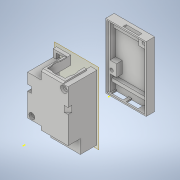
# Autodesk Inventor part: simplemotor
Saved by Autodesk Inventor 2020 (Build 240168000, 168)
## iProperties
Created: 2019-09-09
Part Number: simplemotor
Material: Generic
Document SubType Name: Modeling
Designer: main
Density: 1 g/cm^3
Appearance: Default
Author: main
Autodesk Inventor part; units mm, degrees
ref_plane "YZ Plane" through (0, 0, 0) normal (1, 0, 0) x (0, 1, 0)
ref_plane "XZ Plane" through (0, 0, 0) normal (0, 1, 0) x (-1, 0, 0)
ref_plane "XY Plane" through (0, 0, 0) normal (0, 0, 1) x (1, 0, 0)
sketch "Sketch1" plane through (0, 0, 0) normal (0, 0, 1) x (1, 0, 0)
  line L0 (4.2733, 8.7846) -> (45.3733, 8.7846)
  line L1 (45.3733, 8.7846) -> (45.3733, 74.5846)
  line L2 (45.3733, 74.5846) -> (4.2733, 74.5846)
  line L3 (4.2733, 74.5846) -> (4.2733, 8.7846)
  point P0 (0, 0)
  dimension "d0" = 41.1
  dimension "d1" = 65.8
  constraints: 8 end point, 2 parallel, 1 horizontal, 1 perpendicular
  measures "d0" distance of L1.end L2.end
  measures "d1" distance of L0.end L1.end
extrude "main_body" add sketch "Sketch1" against normal blind 8.6
sketch "Sketch3" plane through (0, 0, 0) normal (0, 0, 1) x (1, 0, 0)
  line L0 (5.5733, 73.2846) -> (44.0733, 73.2846)
  line L1 (44.0733, 73.2846) -> (44.0733, 10.0846)
  line L2 (44.0733, 10.0846) -> (5.5733, 10.0846)
  line L3 (5.5733, 10.0846) -> (5.5733, 73.2846)
  line L4 (4.2733, 74.5846) -> (4.2733, 8.7846) projected
  line L5 (45.3733, 74.5846) -> (4.2733, 74.5846) projected
  line L6 (45.3733, 8.7846) -> (45.3733, 74.5846) projected
  line L7 (4.2733, 8.7846) -> (45.3733, 8.7846) projected
  point P0 (0, 0)
  dimension "d4" = 1.3
  dimension "d5" = 1.3
  dimension "d6" = 1.3
  dimension "d7" = 1.3
  constraints: 8 end point, 2 parallel, 1 horizontal, 1 perpendicular
  measures "d4" distance between parallel lines of L4 L3
  measures "d5" distance between parallel lines of L5 L0
  measures "d6" distance between parallel lines of L6 L1
  measures "d7" distance between parallel lines of L7 L2
extrude "hole_pcb" cut sketch "Sketch3" against normal blind 1.6 contours L0 L1 L2 L3
sketch "Sketch4" plane through (0, 0, -1.6) normal (0, 0, 1) x (1, 0, 0)
  line L0 (7.0733, 73.2846) -> (42.5733, 73.2846)
  line L1 (42.5733, 73.2846) -> (42.5733, 10.0846)
  line L2 (42.5733, 10.0846) -> (7.0733, 10.0846)
  line L3 (7.0733, 10.0846) -> (7.0733, 73.2846)
  line L4 (5.5733, 73.2846) -> (44.0733, 73.2846) projected
  line L5 (44.0733, 10.0846) -> (5.5733, 10.0846) projected
  line L6 (5.5733, 10.0846) -> (5.5733, 73.2846) projected
  line L7 (44.0733, 73.2846) -> (44.0733, 10.0846) projected
  point P0 (0, 0)
  dimension "d10" = 1.5
  dimension "d11" = 1.5
  constraints: 8 end point, 2 collinear, 2 parallel, 1 horizontal, 1 perpendicular
  measures "d10" distance between parallel lines of L6 L3
  measures "d11" distance between parallel lines of L7 L1
extrude "hole_bottom" cut sketch "Sketch4" against normal blind 5.7 contours L0 L1 L2 L3
sketch "Sketch5" plane through (0, 0, -1.6) normal (0, 0, 1) x (1, 0, 0)
  line L0 (13.6943, 26.5086) -> (5.5733, 26.5086)
  line L1 (5.5733, 26.5086) -> (5.5733, 38.5086)
  line L2 (5.5733, 38.5086) -> (13.6943, 38.5086)
  line L3 (13.6943, 38.5086) -> (13.6943, 26.5086)
  line L4 (5.5733, 10.0846) -> (5.5733, 73.2846) projected
  line L5 (44.0733, 10.0846) -> (5.5733, 10.0846) projected
  point P0 (0, 0)
  dimension "d14" = 16.424
  dimension "d15" = 12
  dimension "d16" = 8.121
  constraints: 8 end point, 2 parallel, 1 collinear, 1 horizontal, 1 perpendicular
  measures "d14" distance between parallel lines of L5 L0
  measures "d15" distance of L0.end L1.end
  measures "d16" distance of L1.end L2.end
extrude "support1" add sketch "Sketch5" against normal blind 5.7
sketch "Sketch6" plane through (0, 0, -1.6) normal (0, 0, 1) x (1, 0, 0)
  line L0 (36.4523, 65.6636) -> (44.0733, 65.6636)
  line L1 (44.0733, 65.6636) -> (44.0733, 73.2846)
  line L2 (44.0733, 73.2846) -> (36.4523, 73.2846)
  line L3 (36.4523, 73.2846) -> (36.4523, 65.6636)
  line L4 (5.5733, 73.2846) -> (44.0733, 73.2846) projected
  line L5 (44.0733, 73.2846) -> (44.0733, 10.0846) projected
  point P0 (0, 0)
  dimension "d19" = 7.621
  dimension "d20" = 7.621
  constraints: 8 end point, 2 collinear, 2 parallel, 1 horizontal, 1 perpendicular
  measures "d19" distance of L0.start L0.end
  measures "d20" distance of L2.end L0.start
extrude "support2" add sketch "Sketch6" against normal blind 5.7
sketch "Sketch7" plane through (0, 0, -1.6) normal (0, 0, 1) x (1, 0, 0)
  circle A0 centre (41.2063, 70.3866) radius 1.7
  line L0 (44.0733, 73.2846) -> (44.0733, 10.0846) projected
  line L1 (5.5733, 73.2846) -> (44.0733, 73.2846) projected
  circle A1 centre (8.6943, 30.5086) radius 1.7
  line L2 (5.5733, 10.0846) -> (5.5733, 73.2846) projected
  line L3 (44.0733, 10.0846) -> (5.5733, 10.0846) projected
  point P0 (0, 0)
  dimension "d23" = 2.867
  dimension "d24" = 2.898
  dimension "d25" = 3.4
  dimension "d26" = 3.121
  dimension "d27" = 20.424
  dimension "d28" = 3.4
  constraints: 2 centre point
  measures "d23" distance from line of L0 A0.centre
  measures "d24" distance from line of L1 A0.centre
  measures "d25" diameter of A0
  measures "d26" distance from line of L2 A1.centre
  measures "d27" distance from line of L3 A1.centre
  measures "d28" diameter of A1
sketch "Sketch9" plane through (4.2733, 8.7846, 0) normal (0, -1, 0) x (1, 0, 0)
  line L0 (4.009, -1.6) -> (16.009, -1.6)
  line L1 (16.009, -1.6) -> (16.009, -7.3)
  line L2 (16.009, -7.3) -> (4.009, -7.3)
  line L3 (4.009, -7.3) -> (4.009, -1.6)
  line L4 (0, 0) -> (41.1, 0) projected
  line L5 (1.3, 0) -> (1.3, -1.6) projected
  line L6 (19.249, -1.6) -> (31.249, -1.6)
  line L7 (31.249, -1.6) -> (31.249, -7.3)
  line L8 (31.249, -7.3) -> (19.249, -7.3)
  line L9 (19.249, -7.3) -> (19.249, -1.6)
  point P0 (-4.2733, 0)
  dimension "d35" = 1.6
  dimension "d36" = 5.7
  dimension "d37" = 12
  dimension "d38" = 2.709
  dimension "d39" = 17.949
  constraints: 16 end point, 4 parallel, 3 collinear, 2 horizontal, 2 perpendicular
  measures "d35" distance between parallel lines of L4 L0
  measures "d36" distance of L2.end L0.start
  measures "d37" distance of L1.end L2.end
  measures "d38" distance between parallel lines of L5 L3
  measures "d39" distance between parallel lines of L5 L9
extrude "j1_j2_holes" cut sketch "Sketch9" against normal blind 1.3
sketch "Sketch10" plane through (4.2733, 74.5846, 0) normal (0, 1, 0) x (1, 0, 0)
  line L0 (15.979, 1.6) -> (31.979, 1.6)
  line L1 (31.979, 1.6) -> (31.979, 4.8)
  line L2 (31.979, 4.8) -> (15.979, 4.8)
  line L3 (15.979, 4.8) -> (15.979, 1.6)
  line L4 (16.009, 1.6) -> (4.009, 1.6) projected
  line L5 (1.3, 0) -> (1.3, 1.6) projected
  point P0 (-4.2733, 0)
  dimension "d42" = 3.2
  dimension "d43" = 16
  dimension "d44" = 14.679
  constraints: 8 end point, 2 parallel, 1 collinear, 1 horizontal, 1 perpendicular
  measures "d42" distance of L2.end L0.start
  measures "d43" distance of L1.end L2.end
  measures "d44" distance between parallel lines of L3 L5
extrude "j3_hole" cut sketch "Sketch10" against normal blind 1.3
sketch "Sketch11" plane through (0, 0, -7.3) normal (0, 0, 1) x (1, 0, 0)
  line L0 (7.0733, 18.5846) -> (42.5733, 18.5846)
  line L1 (42.5733, 18.5846) -> (42.5733, 22.0846)
  line L2 (42.5733, 22.0846) -> (7.0733, 22.0846)
  line L3 (7.0733, 22.0846) -> (7.0733, 18.5846)
  line L4 (7.0733, 10.0846) -> (7.0733, 26.5086) projected
  line L5 (42.5733, 65.6636) -> (42.5733, 10.0846) projected
  line L6 (44.0733, 10.0846) -> (5.5733, 10.0846) projected
  point P0 (0, 0)
  dimension "d47" = 8.5
  dimension "d48" = 12
  constraints: 8 end point, 2 collinear, 2 parallel, 1 horizontal, 1 perpendicular
  measures "d47" distance between parallel lines of L0 L6
  measures "d48" distance between parallel lines of L6 L2
extrude "stifness_beam_1" add sketch "Sketch11" along normal blind 3.7 contours L3 L2 L1 L0
sketch "Sketch12" plane through (0, 0, -7.3) normal (0, 0, 1) x (1, 0, 0)
  line L0 (36.4523, 73.2846) -> (7.0733, 73.2846)
  line L1 (7.0733, 73.2846) -> (7.0733, 65.6636)
  line L2 (7.0733, 65.6636) -> (36.4523, 65.6636)
  line L3 (36.4523, 65.6636) -> (36.4523, 73.2846)
  line L4 (36.4523, 73.2846) -> (36.4523, 65.6636) projected
  line L5 (7.0733, 38.5086) -> (7.0733, 73.2846) projected
  line L6 (5.5733, 73.2846) -> (44.0733, 73.2846) projected
  line L7 (36.4523, 65.6636) -> (42.5733, 65.6636) projected
  point P0 (0, 0)
  constraints: 8 end point, 4 collinear, 2 parallel, 1 horizontal, 1 perpendicular
extrude "stifness_beam_2" add sketch "Sketch12" along normal blind 2.5
sketch "Sketch13" plane through (0, 0, -8.6) normal (0, 0, -1) x (-1, 0, 0)
  point P0 (0, 0)
ref_plane "Work Plane1" through (0, 0, 50) normal (0, 0, 1) x (1, 0, 0)
sketch "Sketch15" plane through (0, 0, 50) normal (0, 0, 1) x (1, 0, 0)
  line L0 (45.3733, 74.5846) -> (4.2733, 74.5846)
  line L1 (4.2733, 74.5846) -> (4.2733, 8.7846)
  line L2 (4.2733, 8.7846) -> (45.3733, 8.7846)
  line L3 (45.3733, 8.7846) -> (45.3733, 74.5846)
  line L4 (45.3733, 8.7846) -> (45.3733, 74.5846) projected
  line L5 (45.3733, 74.5846) -> (4.2733, 74.5846) projected
  line L6 (4.2733, 74.5846) -> (4.2733, 8.7846) projected
  line L7 (4.2733, 8.7846) -> (45.3733, 8.7846) projected
  point P0 (0, 0)
  constraints: 8 end point, 4 collinear, 2 parallel, 1 horizontal, 1 perpendicular
extrude "Extrusion12" add sketch "Sketch15" along normal blind 29.3
sketch "Sketch16" plane through (0, 0, 50) normal (0, 0, 1) x (1, 0, 0)
  line L0 (7.0733, 73.2846) -> (42.5733, 73.2846)
  line L1 (42.5733, 73.2846) -> (42.5733, 10.0846)
  line L2 (42.5733, 10.0846) -> (7.0733, 10.0846)
  line L3 (7.0733, 10.0846) -> (7.0733, 73.2846)
  line L4 (7.0733, 10.0846) -> (7.0733, 26.5086) projected
  line L5 (42.5733, 10.0846) -> (35.5223, 10.0846) projected
  line L6 (42.5733, 65.6636) -> (42.5733, 10.0846) projected
  line L7 (7.0733, 73.2846) -> (20.2523, 73.2846) projected
  point P0 (0, 0)
  constraints: 8 end point, 4 collinear, 2 parallel, 1 horizontal, 1 perpendicular
extrude "Extrusion13" cut sketch "Sketch16" along normal blind 28
sketch "Sketch17" plane through (0, 0, 50) normal (0, 0, -1) x (-1, 0, 0)
  line L0 (-42.5733, 27.5846) -> (-44.2733, 27.5846)
  line L1 (-44.2733, 27.5846) -> (-44.2733, 45.2846)
  line L2 (-44.2733, 45.2846) -> (-42.5733, 45.2846)
  line L3 (-42.5733, 45.2846) -> (-42.5733, 27.5846)
  line L4 (-42.5733, 10.0846) -> (-42.5733, 73.2846) projected
  line L5 (-7.0733, 10.0846) -> (-42.5733, 10.0846) projected
  line L6 (-42.5733, 73.2846) -> (-7.0733, 73.2846) projected
  point P0 (0, 0)
  dimension "d68" = 1.7
  dimension "d69" = 17.5
  dimension "d70" = 28
  constraints: 8 end point, 2 parallel, 1 collinear, 1 horizontal, 1 perpendicular
  measures "d68" distance of L0.start L0.end
  measures "d69" distance between parallel lines of L5 L0
  measures "d70" distance between parallel lines of L6 L2
extrude "Extrusion14" cut sketch "Sketch17" against normal blind 28
sketch "Sketch18" plane through (0, 0, 50) normal (0, 0, 1) x (1, 0, 0)
  line L0 (36.4523, 65.6636) -> (42.5733, 65.6636)
  line L1 (42.5733, 65.6636) -> (42.5733, 73.2846)
  line L2 (42.5733, 73.2846) -> (36.4523, 73.2846)
  line L3 (36.4523, 73.2846) -> (36.4523, 65.6636)
  line L4 (42.5733, 73.2846) -> (42.5733, 45.2846) projected
  line L5 (7.0733, 73.2846) -> (42.5733, 73.2846) projected
  line L6 (36.4523, 73.2846) -> (36.4523, 65.6636) projected
  line L7 (36.4523, 65.6636) -> (42.5733, 65.6636) projected
  line L8 (11.7943, 26.5086) -> (7.0733, 26.5086)
  line L9 (7.0733, 26.5086) -> (7.0733, 34.5086)
  line L10 (7.0733, 34.5086) -> (11.7943, 34.5086)
  line L11 (11.7943, 34.5086) -> (11.7943, 26.5086)
  line L12 (7.0733, 10.0846) -> (7.0733, 73.2846) projected
  line L13 (7.0733, 26.5086) -> (13.6943, 26.5086) projected
  circle A0 centre (8.6943, 30.5086) radius 1.6 projected
  point P0 (0, 0)
  dimension "d73" = 4
  dimension "d74" = 3.1
  constraints: 16 end point, 6 collinear, 4 parallel, 2 horizontal, 2 perpendicular
  measures "d73" distance from line of A0.centre L10
  measures "d74" distance from line of L11 A0.centre
extrude "Extrusion15" add sketch "Sketch18" along normal blind 28 contours L3 L2 L1 L0 | L10 L11 L8 L9 | A0
extrude "Extrusion16" cut sketch "Sketch7" along normal blind 100 and the other way blind 10 contours A0 | A1
sketch "Sketch19" plane through (0, 0, -8.6) normal (0, 0, -1) x (-1, 0, 0)
  circle A0 centre (-8.6943, 30.5086) radius 3
  circle A1 centre (-8.6943, 30.5086) radius 1.7 projected
  circle A2 centre (-41.2063, 70.3866) radius 3.5
  circle A3 centre (-41.2063, 70.3866) radius 1.7 projected
  point P0 (0, 0)
  dimension "d81" = 6
  dimension "d82" = 7
  constraints: 2 centre point, 2 concentric
  measures "d81" diameter of A0
  measures "d82" diameter of A2
extrude "Extrusion17" cut sketch "Sketch19" along normal blind 2.5 from surface at -87.9
sketch "Sketch21" plane through (4.2733, 8.7846, 50) normal (0, -1, 0) x (1, 0, 0)
  line L0 (18.479, 1.8) -> (29.479, 1.8)
  line L1 (29.479, 1.8) -> (29.479, 8.6)
  line L2 (29.479, 8.6) -> (18.479, 8.6)
  line L3 (18.479, 8.6) -> (18.479, 1.8)
  line L4 (0, 0) -> (41.1, 0) projected
  line L5 (1.3, -50) -> (1.3, -51.6) projected
  point P0 (-4.2733, -50)
  dimension "d92" = 1.8
  dimension "d93" = 6.8
  dimension "d94" = 11
  dimension "d95" = 17.179
  constraints: 8 end point, 2 parallel, 1 horizontal, 1 perpendicular
  measures "d92" distance between parallel lines of L4 L0
  measures "d93" distance of L2.end L0.start
  measures "d94" distance of L1.end L2.end
  measures "d95" distance between parallel lines of L3 L5
extrude "Extrusion19" cut sketch "Sketch21" against normal blind 1.3
sketch "Sketch22" plane through (0, 0, -7.3) normal (0, 0, 1) x (1, 0, 0)
  point P0 (0, 0)
sketch "Sketch23" plane through (0, 0, 50) normal (0, 0, 1) x (1, 0, 0)
  point P0 (0, 0)
sketch "Sketch24" plane through (0, 0, 50) normal (0, 0, 1) x (1, 0, 0)
  line L0 (18.8663, 65.5996) -> (4.2733, 65.5996)
  line L1 (4.2733, 65.5996) -> (4.2733, 74.5846)
  line L2 (4.2733, 74.5846) -> (18.8663, 74.5846)
  line L3 (18.8663, 74.5846) -> (18.8663, 65.5996)
  line L4 (19.2523, 74.5846) -> (4.2733, 74.5846)
  line L5 (4.2733, 74.5846) -> (4.2733, 8.7846) projected
  line L6 (45.3733, 74.5846) -> (4.2733, 74.5846) projected
  point P0 (0, 0)
  dimension "d98" = 8.985
  dimension "d110" = 14.593
  constraints: 10 end point, 2 collinear, 2 parallel
  measures "d98" distance of L2.end L0.start
  measures "d110" distance between parallel lines of L1 L3
extrude "Extrusion20" add sketch "Sketch24" along normal blind 29.3
sketch "Sketch20" plane through (4.2733, 74.5846, 50) normal (0, 1, 0) x (1, 0, 0)
  line L0 (32.979, -5.7) -> (14.979, -5.7)
  line L1 (14.979, -5.7) -> (14.979, 0)
  line L2 (14.979, 0) -> (32.979, 0)
  line L3 (32.979, 0) -> (32.979, -5.7)
  line L4 (41.1, 0) -> (0, 0) projected
  line L5 (41.1, 0) -> (41.1, -29.3) projected
  line L6 (1.3, 50) -> (1.3, 51.6) projected
  point P0 (-4.2733, 50)
  dimension "d86" = 18
  dimension "d88" = 13.679
  dimension "d89" = 5.7
  constraints: 8 end point, 2 parallel, 1 collinear, 1 horizontal, 1 perpendicular
  measures "d86" distance of L0.start L0.end
  measures "d88" distance between parallel lines of L1 L6
  measures "d89" distance of L2.end L0.start
extrude "Extrusion18" cut sketch "Sketch20" against normal blind 12
sketch "Sketch25" plane through (0, 0, 79.3) normal (0, 0, 1) x (1, 0, 0)
  line L0 (18.2163, 66.8996) -> (4.2733, 66.8996)
  line L1 (4.2733, 66.8996) -> (4.2733, 74.5846)
  line L2 (4.2733, 74.5846) -> (18.2163, 74.5846)
  line L3 (18.2163, 74.5846) -> (18.2163, 66.8996)
  line L4 (4.2733, 74.5846) -> (4.2733, 65.6496) projected
  line L5 (19.8663, 74.5846) -> (4.2733, 74.5846) projected
  line L6 (5.5733, 10.0846) -> (5.5733, 73.2846) projected
  line L7 (5.5733, 73.2846) -> (44.0733, 73.2846) projected
  point P0 (0, 0)
  dimension "d101" = 12.643
  dimension "d102" = 6.385
  constraints: 8 end point, 2 collinear, 2 parallel, 1 horizontal, 1 perpendicular
  measures "d101" distance between parallel lines of L6 L3
  measures "d102" distance between parallel lines of L7 L0
extrude "Extrusion21" cut sketch "Sketch25" against normal blind 25.9
sketch "Sketch26" plane through (0, 0, 53.4) normal (0, 0, 1) x (1, 0, 0)
  line L0 (18.2163, 66.8996) -> (7.5163, 66.8996)
  line L1 (7.5163, 66.8996) -> (7.5163, 72.3496)
  line L2 (7.5163, 72.3496) -> (18.2163, 72.3496)
  line L3 (18.2163, 72.3496) -> (18.2163, 66.8996)
  line L4 (18.2163, 66.8996) -> (4.2733, 66.8996) projected
  line L5 (18.2163, 74.5846) -> (18.2163, 66.8996) projected
  point P0 (0, 0)
  dimension "d105" = 5.45
  dimension "d106" = 10.7
  constraints: 8 end point, 2 collinear, 2 parallel, 1 horizontal, 1 perpendicular
  measures "d105" distance of L0.end L1.end
  measures "d106" distance of L1.end L2.end
extrude "Extrusion22" cut sketch "Sketch26" against normal blind 3.4
sketch "Sketch27" plane through (0, 0, 50) normal (0, 0, 1) x (1, 0, 0)
  line L0 (18.8663, 27.2796) -> (7.0733, 27.2796)
  line L1 (7.0733, 27.2796) -> (7.0733, 10.0846)
  line L2 (7.0733, 10.0846) -> (18.8663, 10.0846)
  line L3 (18.8663, 10.0846) -> (18.8663, 27.2796)
  line L4 (7.0733, 10.0846) -> (7.0733, 26.5086) projected
  line L5 (42.5733, 10.0846) -> (7.0733, 10.0846) projected
  line L6 (5.5733, 10.0846) -> (5.5733, 73.2846) projected
  point P0 (0, 0)
  dimension "d111" = 17.195
  dimension "d112" = 13.293
  constraints: 8 end point, 2 collinear, 2 parallel, 1 horizontal, 1 perpendicular
  measures "d111" distance between parallel lines of L2 L0
  measures "d112" distance between parallel lines of L6 L3
extrude "Extrusion23" add sketch "Sketch27" along normal blind 29.3
sketch "Sketch28" plane through (0, 0, 79.3) normal (0, 0, 1) x (1, 0, 0)
  point P0 (0, 0)
sketch "Sketch29" plane through (0, 0, 79.3) normal (0, 0, 1) x (1, 0, 0)
  line L0 (18.2163, 26.6296) -> (4.2733, 26.6296)
  line L1 (4.2733, 26.6296) -> (4.2733, 8.7846)
  line L2 (4.2733, 8.7846) -> (18.2163, 8.7846)
  line L3 (18.2163, 8.7846) -> (18.2163, 26.6296)
  line L4 (4.2733, 66.8996) -> (4.2733, 8.7846) projected
  line L5 (4.2733, 8.7846) -> (45.3733, 8.7846) projected
  line L6 (18.8663, 27.2796) -> (11.7943, 27.2796) projected
  line L7 (18.8663, 10.0846) -> (18.8663, 27.2796) projected
  point P0 (0, 0)
  dimension "d169" = 0.65
  dimension "d170" = 0.65
  constraints: 8 end point, 2 collinear, 2 parallel, 1 horizontal, 1 perpendicular
  measures "d169" distance between parallel lines of L6 L0
  measures "d170" distance between parallel lines of L7 L3
extrude "Extrusion24" cut sketch "Sketch29" against normal blind 25.9
sketch "Sketch30" plane through (0, 0, 53.4) normal (0, 0, 1) x (1, 0, 0)
  point P0 (0, 0)
sketch "Sketch31" plane through (0, 0, 53.4) normal (0, 0, 1) x (1, 0, 0)
  line L0 (7.5163, 21.1796) -> (18.2163, 21.1796)
  line L1 (18.2163, 21.1796) -> (18.2163, 26.6296)
  line L2 (18.2163, 26.6296) -> (7.5163, 26.6296)
  line L3 (7.5163, 26.6296) -> (7.5163, 21.1796)
  line L4 (4.2733, 26.6296) -> (18.2163, 26.6296) projected
  line L5 (18.2163, 26.6296) -> (18.2163, 8.7846) projected
  point P0 (0, 0)
  point P1 (7.0733, 26.5796)
  point P2 (18.5663, 10.0846)
  point P3 (18.2163, 8.7846)
  dimension "d119" = 5.45
  dimension "d120" = 10.7
  constraints: 8 end point, 2 horizontal, 2 parallel, 1 perpendicular, 1 vertical, 2 other
  measures "d119" distance of L2.end L0.start
  measures "d120" distance of L0.start L0.end
extrude "Extrusion25" cut sketch "Sketch31" against normal blind 3.4
sketch "Sketch33" plane through (18.8663, 10.0846, 50) normal (1, 0, 0) x (0, 0, -1)
  line L0 (-29.3, 17.145) -> (-24.3, 17.145)
  line L1 (-24.3, 17.145) -> (-24.3, 12.145)
  line L2 (-24.3, 12.145) -> (-29.3, 12.145)
  line L3 (-29.3, 12.145) -> (-29.3, 17.145)
  line L4 (-29.3, 0) -> (-29.3, 17.145) projected
  line L5 (-7, 17.145) -> (-28, 17.145) projected
  point P0 (50, -10.0846)
  dimension "d126" = 5
  dimension "d127" = 5
  constraints: 8 end point, 2 collinear, 2 parallel, 1 horizontal, 1 perpendicular
  measures "d126" distance of L1.end L2.end
  measures "d127" distance of L0.end L1.end
extrude "Extrusion27" add sketch "Sketch33" along normal blind 24.557
sketch "Sketch34" plane through (18.8663, 10.0846, 50) normal (1, 0, 0) x (0, 0, -1)
  line L0 (0, 17.195) -> (-28, 17.195)
  line L1 (-28, 17.195) -> (-28, 17.145)
  line L2 (-28, 17.145) -> (0, 17.145)
  line L3 (0, 17.145) -> (0, 17.195)
  line L4 (0, 17.195) -> (-28, 17.195) projected
  line L5 (0, 0) -> (0, 17.195) projected
  line L6 (-28, 17.145) -> (-24.3, 17.145) projected
  line L7 (-28, 17.145) -> (-28, 17.195) projected
  point P0 (50, -10.0846)
  constraints: 8 end point, 4 collinear, 2 parallel, 1 horizontal, 1 perpendicular
extrude "Extrusion28" cut sketch "Sketch34" against normal up to surface (7.072 mm away)
sketch "Sketch35" plane through (0, 0, 79.3) normal (0, 0, 1) x (1, 0, 0)
  point P0 (0, 0)
sketch "Sketch36" plane through (0, 0, 79.3) normal (0, 0, 1) x (1, 0, 0)
  point P0 (0, 0)
sketch "Sketch37" plane through (0, 0, 79.3) normal (0, 0, 1) x (1, 0, 0)
  line L0 (6.9912, 27.5586) -> (5.288, 30.5086)
  line L1 (5.288, 30.5086) -> (6.9912, 33.4586)
  line L2 (6.9912, 33.4586) -> (10.3975, 33.4586)
  line L3 (10.3975, 33.4586) -> (12.1007, 30.5086)
  line L4 (12.1007, 30.5086) -> (10.3975, 27.5586)
  line L5 (10.3975, 27.5586) -> (6.9912, 27.5586)
  line L6 (4.2733, 26.6296) -> (18.2163, 26.6296) projected
  circle A0 centre (8.6943, 30.5086) radius 2.95 construction
  circle A1 centre (8.6943, 30.5086) radius 1.7 projected
  line L7 (39.5032, 67.4366) -> (37.8, 70.3866)
  line L8 (37.8, 70.3866) -> (39.5032, 73.3366)
  line L9 (39.5032, 73.3366) -> (42.9095, 73.3366)
  line L10 (42.9095, 73.3366) -> (44.6127, 70.3866)
  line L11 (44.6127, 70.3866) -> (42.9095, 67.4366)
  line L12 (42.9095, 67.4366) -> (39.5032, 67.4366)
  line L13 (45.3733, 74.5846) -> (18.2163, 74.5846) projected
  circle A2 centre (41.2063, 70.3866) radius 2.95 construction
  circle A3 centre (41.2063, 70.3866) radius 1.7 projected
  point P0 (0, 0)
  point P1 (8.6943, 30.5086)
  point P2 (19.1163, 26.5796)
  dimension "d132" = 5.9
  dimension "d133" = 5.9
  constraints: 24 end point, 6 tangent, 2 centre point, 2 concentric, 1 horizontal, 1 parallel, 27 other
  measures "d132" distance between parallel lines of L2 L5
  measures "d133" distance between parallel lines of L9 L12
extrude "Extrusion29" cut sketch "Sketch37" along normal blind 3 from surface at -87.9
chamfer "Chamfer2" distance 7 angle 45 2 edges at (39.5128, 65.6636, 78) (36.4523, 69.4741, 78)
sketch "Sketch38" plane through (42.5733, 45.2846, 50) normal (-1, 0, 0) x (0, 0, 1)
  line L0 (28, 0) -> (24, 0)
  line L1 (24, 0) -> (24, 5)
  line L2 (24, 5) -> (28, 5)
  line L3 (28, 5) -> (28, 0)
  line L4 (0, 0) -> (28, 0) projected
  line L5 (28, 0) -> (28, 13.379) projected
  point P0 (-50, -45.2846)
  dimension "d142" = 5
  dimension "d143" = 4
  constraints: 8 end point, 2 collinear, 2 parallel, 1 horizontal, 1 perpendicular
  measures "d142" distance of L0.end L1.end
  measures "d143" distance of L1.end L2.end
extrude "Extrusion30" add sketch "Sketch38" along normal blind 35.5
sketch "Sketch39" plane through (7.0733, 34.5086, 50) normal (0, 1, 0) x (1, 0, 0)
  line L0 (0, -24) -> (4.721, -24)
  line L1 (4.721, -24) -> (4.721, -28)
  line L2 (4.721, -28) -> (0, -28)
  line L3 (0, -28) -> (0, -24)
  line L4 (4.721, 0) -> (4.721, -28) projected
  line L5 (0, -28) -> (0, 0) projected
  line L6 (4.721, -28) -> (0, -28) projected
  point P0 (-7.0733, 50)
  dimension "d146" = 4
  constraints: 8 end point, 3 collinear, 2 parallel, 1 horizontal, 1 perpendicular
  measures "d146" distance of L0.end L1.end
extrude "Extrusion31" add sketch "Sketch39" along normal blind 32
sketch "Sketch40" plane through (11.7943, 27.2296, 78) normal (1, 0, 0) x (0, 0, -1)
  line L0 (0, 0) -> (0, 6)
  line L1 (0, 6) -> (6, 0)
  line L2 (6, 0) -> (0, 0)
  line L3 (0, 0) -> (0, 18.055) projected
  line L4 (28, 0) -> (0, 0) projected
  point P0 (78, -27.2296)
  point P1 (0, 0.05)
  dimension "d149" = 6
  dimension "d150" = 6
  constraints: 6 end point, 2 collinear
  measures "d149" distance of L0.start L0.end
  measures "d150" distance of L1.end L0.start
extrude "Extrusion32" add sketch "Sketch40" along normal up to surface (7.072 mm away)
sketch "Sketch41" plane through (0, 0, 78) normal (0, 0, -1) x (-1, 0, 0)
  point P0 (0, 0)
sketch "Sketch42" plane through (0, 0, 78) normal (0, 0, -1) x (-1, 0, 0)
  point P0 (0, 0)
sketch "Sketch43" plane through (0, 0, 78) normal (0, 0, -1) x (-1, 0, 0)
  point P0 (0, 0)
sketch "Sketch44" plane through (0, 0, 78) normal (0, 0, -1) x (-1, 0, 0)
  line L0 (-20.3663, 10.0846) -> (-18.8663, 10.0846)
  line L1 (-18.8663, 10.0846) -> (-18.8663, 27.2296)
  line L2 (-18.8663, 27.2296) -> (-20.3663, 27.2296)
  line L3 (-20.3663, 27.2296) -> (-20.3663, 10.0846)
  line L4 (-18.8663, 27.2296) -> (-18.8663, 33.2296) projected
  line L5 (-18.8663, 10.0846) -> (-42.5733, 10.0846) projected
  line L6 (-11.7943, 27.2296) -> (-18.8663, 27.2296) projected
  point P0 (0, 0)
  point P1 (-18.8663, 22.2296)
  point P2 (-19.2163, 10.0846)
  point P3 (-18.2163, 27.2296)
  dimension "d153" = 1.5
  constraints: 8 end point, 3 collinear, 2 parallel, 1 horizontal, 1 perpendicular
  measures "d153" distance between parallel lines of L3 L1
extrude "Extrusion33" add sketch "Sketch44" along normal blind 12
sketch "Sketch45" plane through (0, 0, 53.4) normal (0, 0, 1) x (1, 0, 0)
  line L0 (18.2163, 21.1796) -> (18.2163, 8.7846)
  line L1 (18.2163, 8.7846) -> (15.2163, 8.7846)
  line L2 (15.2163, 8.7846) -> (18.2163, 21.1796)
  line L3 (18.2163, 8.7846) -> (4.2733, 8.7846) projected
  line L4 (18.2163, 21.1796) -> (18.2163, 8.7846) projected
  line L5 (18.2163, 21.1796) -> (7.5163, 21.1796) projected
  point P0 (0, 0)
  point P1 (19.2163, 10.0846)
  point P2 (19.1163, 21.1296)
  dimension "d156" = 3
  constraints: 4 end point, 1 collinear, 6 other
  measures "d156" distance of L1.start L1.end
extrude "Extrusion34" add sketch "Sketch45" along normal up to surface (25.9 mm away)
sketch "Sketch46" plane through (0, 0, 50) normal (0, 0, -1) x (-1, 0, 0)
  line L0 (-42.5733, 27.5846) -> (-42.9733, 27.5846)
  line L1 (-42.9733, 27.5846) -> (-42.9733, 10.0846)
  line L2 (-42.9733, 10.0846) -> (-42.5733, 10.0846)
  line L3 (-42.5733, 10.0846) -> (-42.5733, 27.5846)
  line L4 (-42.5733, 10.0846) -> (-42.5733, 27.5846) projected
  line L5 (-42.5733, 27.5846) -> (-44.2733, 27.5846) projected
  line L6 (-18.8663, 10.0846) -> (-42.5733, 10.0846) projected
  point P0 (0, 0)
  dimension "d159" = 0.4
  constraints: 8 end point, 3 collinear, 2 parallel, 1 horizontal, 1 perpendicular
  measures "d159" distance between parallel lines of L3 L1
extrude "Extrusion35" cut sketch "Sketch46" against normal blind 16
sketch "Sketch47" plane through (42.5733, 50.2846, 78) normal (0, 1, 0) x (1, 0, 0)
  line L0 (0, 4) -> (-4, 4)
  line L1 (-4, 4) -> (-4, 0)
  line L2 (-4, 0) -> (0, 0)
  line L3 (0, 0) -> (0, 4)
  line L4 (0, 4) -> (0, 0) projected
  line L5 (0, 0) -> (-30.779, 0) projected
  line L6 (0, 4) -> (-30.779, 4) projected
  point P0 (-42.5733, 78)
  constraints: 8 end point, 3 collinear, 2 parallel, 2 perpendicular, 1 horizontal
extrude "Extrusion36" add sketch "Sketch47" along normal up to surface (15.379 mm away)
sketch "Sketch48" plane through (44.9733, 50.2846, 79.3) normal (0, 1, 0) x (1, 0, 0)
  line L0 (0.4, 4) -> (0.4, 0)
  line L1 (0.4, 0) -> (-3.6, 0)
  line L2 (-3.6, 0) -> (0.4, 4)
  line L3 (0.4, 0) -> (-26.757, 0) projected
  line L4 (0.4, 29.3) -> (0.4, 0) projected
  line L5 (-26.757, 0) -> (-40.7, 0) projected
  line L6 (-40.7, 0) -> (-40.7, 25.9) projected
  line L7 (-36.7, 0) -> (-40.7, 4)
  line L8 (-40.7, 4) -> (-40.7, 0)
  line L9 (-40.7, 0) -> (-36.7, 0)
  point P0 (-44.9733, 79.3)
  point P1 (-36.7, 0)
  dimension "d164" = 4
  constraints: 12 end point, 4 collinear, 3 perpendicular
  measures "d164" distance of L0.end L1.end
extrude "Extrusion38" cut sketch "Sketch48" along normal blind 6
sketch "Sketch49" plane through (20.3663, 10.0846, 78) normal (0, 1, 0) x (1, 0, 0)
  line L0 (22.607, 0) -> (-1.5, 0)
  line L1 (-1.5, 0) -> (-1.5, 12.5)
  line L2 (-1.5, 12.5) -> (22.607, 12.5)
  line L3 (22.607, 12.5) -> (22.607, 0)
  line L4 (22.607, 28) -> (22.607, 12) projected
  line L5 (-1.5, 28) -> (-1.5, 12) projected
  line L6 (-1.5, 28) -> (22.607, 28) projected
  line L7 (0, 0) -> (22.207, 0) projected
  point P0 (-20.3663, 78)
  dimension "d171" = 15.5
  constraints: 8 end point, 3 collinear, 2 parallel, 1 horizontal, 1 perpendicular
  measures "d171" distance between parallel lines of L6 L2
extrude "Extrusion39" add sketch "Sketch49" along normal blind 14 from surface at 0 contours L0 L1 L2 L3
sketch "Sketch52" plane through (4.2733, 8.7846, 50) normal (0, -1, 0) x (1, 0, 0)
  line L0 (10.943, 29.3) -> (41.1, 29.3)
  line L1 (41.1, 29.3) -> (41.1, 16.8)
  line L2 (41.1, 16.8) -> (10.943, 16.8)
  line L3 (10.943, 16.8) -> (10.943, 29.3)
  line L4 (10.943, 29.3) -> (41.1, 29.3) projected
  line L5 (10.943, 3.4) -> (10.943, 29.3) projected
  line L6 (41.1, 0) -> (41.1, 29.3) projected
  line L7 (14.593, 15.5) -> (38.7, 15.5) projected
  point P0 (-4.2733, -50)
  dimension "d177" = 1.3
  constraints: 8 end point, 3 collinear, 2 parallel, 1 horizontal, 1 perpendicular
  measures "d177" distance between parallel lines of L7 L2
extrude "Extrusion40" cut sketch "Sketch52" against normal blind 14
sketch "Sketch53" plane through (45.3733, 74.5846, 79.3) normal (0, 1, 0) x (1, 0, 0)
  line L0 (-26.507, 29.3) -> (-6.207, 29.3)
  line L1 (-6.207, 29.3) -> (-6.207, 3.3)
  line L2 (-6.207, 3.3) -> (-26.507, 3.3)
  line L3 (-26.507, 3.3) -> (-26.507, 29.3)
  line L4 (-26.507, 29.3) -> (-26.507, 1.3) projected
  line L5 (-26.121, 29.3) -> (-41.1, 29.3) projected
  line L6 (-8.121, 23.6) -> (-26.121, 23.6) projected
  point P0 (-45.3733, 79.3)
  dimension "fan_a" = 20.3
  dimension "d181" = 20.3
  constraints: 8 end point, 2 collinear, 2 parallel, 1 horizontal, 1 perpendicular
  measures "fan_a" distance of L1.end L2.end
  measures "d181" distance between parallel lines of L2 L6
extrude "Extrusion41" cut sketch "Sketch53" against normal blind 10
sketch "Sketch54" plane through (45.3733, 74.5846, 79.3) normal (0, 1, 0) x (1, 0, 0)
  line L0 (-4.707, 23.6) -> (-4.707, 1.8)
  line L1 (-4.707, 1.8) -> (-27.157, 1.8)
  line L2 (-27.157, 1.8) -> (-27.157, 23.6)
  line L3 (-27.157, 23.6) -> (-26.507, 23.6)
  line L4 (-26.507, 23.6) -> (-26.507, 3.3)
  line L5 (-26.507, 3.3) -> (-6.207, 3.3)
  line L6 (-6.207, 3.3) -> (-6.207, 23.6)
  line L7 (-6.207, 23.6) -> (-4.707, 23.6)
  line L8 (-27.157, 25.9) -> (-27.157, 0) projected
  line L9 (-26.507, 3.3) -> (-26.507, 29.3) projected
  line L10 (-6.207, 3.3) -> (-26.507, 3.3) projected
  line L11 (-6.207, 29.3) -> (-6.207, 3.3) projected
  point P0 (-45.3733, 79.3)
  dimension "fan_mount_margin" = 1.5
  dimension "d185" = 1.5
  dimension "d186" = 20.3
  dimension "d187" = 20.3
  constraints: 16 end point, 4 collinear, 4 parallel
  measures "fan_mount_margin" distance between parallel lines of L5 L1
  measures "d185" distance between parallel lines of L6 L0
  measures "d186" distance between parallel lines of L7 L5
  measures "d187" distance between parallel lines of L3 L5
extrude "Extrusion42" add sketch "Sketch54" along normal blind 1.5
sketch "Sketch55" plane through (45.3733, 76.0846, 79.3) normal (0, 1, 0) x (1, 0, 0)
  line L0 (-6.207, 3.3) -> (-26.507, 3.3)
  line L1 (-26.507, 3.3) -> (-26.507, 23.6)
  line L2 (-26.507, 23.6) -> (-6.207, 23.6)
  line L3 (-6.207, 23.6) -> (-6.207, 3.3)
  line L4 (-6.207, 23.6) -> (-6.207, 3.3) projected
  line L5 (-4.707, 23.6) -> (-6.207, 23.6) projected
  line L6 (-6.207, 3.3) -> (-26.507, 3.3) projected
  line L7 (-26.507, 3.3) -> (-26.507, 23.6) projected
  point P0 (-45.3733, 79.3)
  constraints: 8 end point, 4 collinear, 2 parallel, 1 horizontal, 1 perpendicular
extrude "Extrusion43" add sketch "Sketch55" against normal blind 1
sketch "Sketch56" plane through (45.3733, 76.0846, 79.3) normal (0, 1, 0) x (1, 0, 0)
  circle A0 centre (-16.357, 13.45) radius 10.15
  line L0 (-6.207, 29.3) -> (-6.207, 23.6) projected
  line L1 (-26.507, 3.3) -> (-6.207, 3.3) projected
  point P0 (-45.3733, 79.3)
  dimension "d192" = 20.3
  constraints: 2 tangent, 1 centre point
  measures "d192" diameter of A0
extrude "Extrusion44" cut sketch "Sketch56" against normal blind 1
sketch "Sketch57" plane through (45.3733, 76.0846, 79.3) normal (0, 1, 0) x (1, 0, 0)
  line L0 (-7.207, 23.6) -> (-25.507, 23.6)
  line L1 (-25.507, 23.6) -> (-25.507, 4.3)
  line L2 (-25.507, 4.3) -> (-7.207, 4.3)
  line L3 (-7.207, 4.3) -> (-7.207, 23.6)
  line L4 (-4.707, 23.6) -> (-16.357, 23.6) projected
  line L5 (-26.507, 3.3) -> (-16.357, 3.3) projected
  line L6 (-26.507, 13.45) -> (-26.507, 3.3) projected
  line L7 (-6.207, 13.45) -> (-6.207, 23.6) projected
  point P0 (-45.3733, 79.3)
  dimension "fan_margin" = 1
  dimension "d196" = 1
  dimension "d198" = 1
  constraints: 8 end point, 2 parallel, 1 collinear, 1 horizontal, 1 perpendicular
  measures "fan_margin" distance between parallel lines of L5 L2
  measures "d196" distance between parallel lines of L6 L1
  measures "d198" distance between parallel lines of L7 L3
extrude "Extrusion45" cut sketch "Sketch57" against normal blind 1
sketch "Sketch58" plane through (40.6663, 74.5846, 77.5) normal (1, 0, 0) x (0, 0, -1)
  line L0 (0, 1.5) -> (-1.8, 0)
  line L1 (-1.8, 0) -> (0, 0)
  line L2 (0, 0) -> (0, 1.5)
  line L3 (0, 0) -> (0, 1.5) projected
  line L4 (27.5, 0) -> (-1.8, 0) projected
  point P0 (77.5, -74.5846)
  constraints: 6 end point, 3 collinear
extrude "Extrusion46" add sketch "Sketch58" against normal up to surface (22.45 mm away)
sketch "Sketch59" plane through (4.2733, 22.7846, 50) normal (0, -1, 0) x (1, 0, 0)
  line L0 (34.6927, 25.6404) -> (20.3423, 25.6404)
  line L1 (20.3423, 25.6404) -> (20.3423, 27.1864)
  line L2 (20.3423, 27.1864) -> (34.6927, 27.1864)
  line L3 (34.6927, 27.1864) -> (34.6927, 25.6404)
  line L4 (20.3423, 24.1864) -> (34.6927, 24.1864)
  line L5 (20.3423, 22.6404) -> (20.3423, 24.1864)
  line L6 (34.6927, 22.6404) -> (20.3423, 22.6404)
  line L7 (34.6927, 24.1864) -> (34.6927, 22.6404)
  line L8 (20.3423, 21.1864) -> (34.6927, 21.1864)
  line L9 (20.3423, 19.6404) -> (20.3423, 21.1864)
  line L10 (34.6927, 19.6404) -> (20.3423, 19.6404)
  line L11 (34.6927, 21.1864) -> (34.6927, 19.6404)
  point P0 (-4.2733, -50)
  dimension "d205" = 3
  constraints: 24 end point, 2 parallel, 1 collinear, 1 horizontal, 1 perpendicular, 1 vertical, 15 other
  measures "d205" distance of L1.end L4.start
extrude "Extrusion47" cut sketch "Sketch59" against normal blind 6
equation "\"d0\" = pcb_w + 2 * d"
equation "\"d1\" = pcb_h + 2 * d"
equation "\"d2\" = d + h_bottom + pcb_d"
equation "\"d4\" = d"
equation "\"d5\" = d"
equation "\"d6\" = d"
equation "\"d7\" = d"
equation "\"d8\" = pcb_d"
equation "\"d10\" = pcb_supp"
equation "\"d11\" = pcb_supp"
equation "\"d12\" = h_bottom"
equation "\"d17\" = h_bottom"
equation "\"d21\" = h_bottom"
equation "\"d23\" = x2"
equation "\"d24\" = y2"
equation "\"d26\" = x1"
equation "\"d27\" = y1"
equation "\"d35\" = pcb_d"
equation "\"d36\" = h_bottom"
equation "\"d40\" = d"
equation "\"d45\" = d"
equation "\"d64\" = h_top + d"
equation "\"d66\" = h_top"
equation "\"d71\" = h_top"
equation "\"d75\" = h_top"
equation "\"d96\" = d"
equation "\"d110\" = 1.5 * d + xt_x + 0.5 * xt_h"
equation "\"d99\" = h_top + d"
equation "\"d89\" = h_bottom"
equation "\"d101\" = xt_x + 0.5 * xt_h"
equation "\"d102\" = xt_2 + 0.5 * xt_w"
equation "\"d105\" = xt_w"
equation "\"d106\" = xt_h"
equation "\"d111\" = 0.5 * xt_w + xt_1 + 0.5 * d"
equation "\"d112\" = 0.5 * xt_h + xt_x + 0.5 * d"
equation "\"d113\" = h_top + d"
equation "\"d169\" = 0.5 * d"
equation "\"d170\" = 0.5 * d"
equation "\"d119\" = xt_w"
equation "\"d120\" = xt_h"
equation "\"d128\" = -0.5 * xt_h + pcb_w - xt_x - d"
equation "\"d144\" = pcb_w - 2 * pcb_supp"
equation "\"pcb_d\" = 1.6"
equation "\"pcb_w\" = 38.5"
equation "\"pcb_h\" = 63.2"
equation "\"h_top\" = 28"
equation "\"h_top_min\" = 21"
equation "\"h_bottom\" = 5.7"
equation "\"d\" = 1.3"
equation "\"pcb_supp\" = 1.5"
equation "\"nucleo\" = 1"
equation "\"xt_w\" = 5.45"
equation "\"xt_h\" = 10.7"
equation "\"x2\" = 2.867"
equation "\"y2\" = 2.898"
equation "\"x1\" = 3.121"
equation "\"y1\" = 20.424"
equation "\"xt_x\" = 7.293"
equation "\"xt_2\" = 3.66"
equation "\"xt_1\" = 13.82"
body "Solid1"
